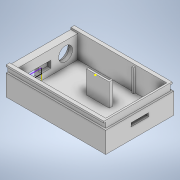
# Autodesk Inventor part: CajaArduinoNano
Saved by Autodesk Inventor 2021 (Build 250183000, 183)
## iProperties
Created: 2020-09-05
Part Number: CajaArduinoNano
Material: Genérico
Document SubType Name: Modeling
Designer: igtw1
Density: 1 g/cm^3
Appearance: Valor por defecto
Author: igtw1
Autodesk Inventor part; units mm, degrees
ref_plane "YZ Plane" through (0, 0, 0) normal (1, 0, 0) x (0, 1, 0)
ref_plane "XZ Plane" through (0, 0, 0) normal (0, 1, 0) x (-1, 0, 0)
ref_plane "XY Plane" through (0, 0, 0) normal (0, 0, 1) x (1, 0, 0)
sketch "Boceto1" plane through (0, 0, 0) normal (0, 1, 0) x (-1, 0, 0)
  line L0 (27.5, -17.5) -> (-27.5, -17.5)
  line L1 (-27.5, -17.5) -> (-27.5, 17.5)
  line L2 (-27.5, 17.5) -> (27.5, 17.5)
  line L3 (27.5, 17.5) -> (27.5, -17.5)
  line L4 (27.5, -17.5) -> (-27.5, 17.5) construction
  line L5 (-27.5, -17.5) -> (27.5, 17.5) construction
  point P0 (0, 0)
  dimension "d0" = 55
  dimension "d1" = 35
  constraints: 12 end point, 2 midpoint, 2 parallel, 1 horizontal, 1 perpendicular
  measures "d0" distance of L1.end L2.end
  measures "d1" distance of L0.end L1.end
extrude "Extrusión1" add sketch "Boceto1" along normal blind 15
sketch "Boceto2" plane through (0, 15, 0) normal (0, 1, 0) x (1, 0, 0)
  line L0 (25.5, -15.5) -> (-25.5, -15.5)
  line L1 (-25.5, -15.5) -> (-25.5, 15.5)
  line L2 (-25.5, 15.5) -> (25.5, 15.5)
  line L3 (25.5, 15.5) -> (25.5, -15.5)
  line L4 (25.5, -15.5) -> (-25.5, 15.5) construction
  line L5 (-25.5, -15.5) -> (25.5, 15.5) construction
  point P0 (0, 0)
  dimension "d4" = 51
  dimension "d5" = 31
  constraints: 12 end point, 2 midpoint, 2 parallel, 1 horizontal, 1 perpendicular
  measures "d4" distance of L1.end L2.end
  measures "d5" distance of L0.end L1.end
extrude "Extrusión2" cut sketch "Boceto2" against normal blind 13
sketch "Boceto3" plane through (-27.5, 0, -17.5) normal (-1, 0, 0) x (0, 0, 1)
  point P0 (17.5, 0)
sketch "Boceto4" plane through (0, 15, 0) normal (0, 1, 0) x (1, 0, 0)
  line L0 (-27.5, 17.5) -> (-27.5, -17.5) projected
  line L1 (-27.5, -17.5) -> (-29.5, -17.5)
  line L2 (-29.5, -17.5) -> (-29.5, 17.5)
  line L3 (-29.5, 17.5) -> (-27.5, 17.5)
  line L4 (-27.5, 17.5) -> (-27.5, -17.5)
  point P0 (0, 0)
  dimension "d8" = 2
  constraints: 8 end point, 2 parallel, 1 horizontal, 1 perpendicular
  measures "d8" distance of L2.end L3.end
extrude "Extrusión3" add sketch "Boceto4" against normal blind 15
sketch "Boceto5" plane through (-29.5, 15, -17.5) normal (-1, 0, 0) x (0, 0, 1)
  line L0 (35, 0) -> (0, 0) projected
  line L1 (0, 0) -> (9, 0)
  line L2 (9, 0) -> (9, -6.5)
  line L3 (2, -13) -> (33, -13) projected
  circle A0 centre (9, -6.5) radius 5.5
  point P0 (17.5, -15)
  dimension "d11" = 9
  dimension "d12" = 6.5
  dimension "d13" = 11
  constraints: 4 end point, 1 centre point, 1 coincident, 1 perpendicular, 1 point on line
  measures "d11" distance of L0.end L1.end
  measures "d12" distance of L1.end L2.end
  measures "d13" diameter of A0
extrude "Extrusión4" cut sketch "Boceto5" against normal blind 2
sketch "Boceto6" plane through (-27.5, 8.5, -8.5) normal (-1, 0, 0) x (0, 0, 1)
  circle A0 centre (0, 0) radius 4
  point P0 (8.5, -8.5)
  dimension "d16" = 8
  constraints: 1 centre point
  measures "d16" diameter of A0
extrude "Extrusión5" cut sketch "Boceto6" against normal blind 2
sketch "Boceto7" plane through (0, 2, 0) normal (0, 1, 0) x (1, 0, 0)
  line L0 (-27.5, 3) -> (-27.5, 14) projected
  line L1 (-27.5, 3) -> (-27.5, 8.5)
  line L2 (-25.5, -15.5) -> (-25.5, 15.5) projected
  line L3 (-25.5, 8.5) -> (-25.5, 1.5)
  line L4 (-25.5, 15.5) -> (25.5, 15.5) projected
  line L5 (7.5, 15.5) -> (7.5, 14.5)
  line L6 (7.5, 14.5) -> (6.5, 14.5)
  line L7 (6.5, 14.5) -> (6.5, 15.5)
  line L8 (6.5, 1.5) -> (6.5, 2.5547)
  line L9 (6.5, 2.5547) -> (7.5, 2.5547)
  line L10 (7.5, 2.5547) -> (7.5, 0.5)
  line L11 (7.5, 0.5) -> (-5.5, 0.5)
  line L12 (-5.5, 0.5) -> (-5.5, 1.5)
  line L13 (-5.5, 1.5) -> (6.5, 1.5)
  point P0 (0, 0)
  dimension "d19" = 7
  dimension "d27" = 32
  constraints: 22 end point, 4 point on line, 3 horizontal, 2 perpendicular, 1 midpoint
  measures "d19" distance of L3.start L3.end
  measures "d27" distance of L3.end L8.start
extrude "Extrusión6" add sketch "Boceto7" along normal blind 13 contours L8 L9 L10 L11 L12 L13
sketch "Boceto8" plane through (0, 2, 0) normal (0, 1, 0) x (1, 0, 0)
  line L0 (6.5, 1.5) -> (6.5, 2.5547) projected
  line L1 (-25.5, 15.5) -> (25.5, 15.5) projected
  line L2 (6.5, 15.5) -> (6.5, 14.5)
  line L3 (6.5, 14.5) -> (7.5, 14.5)
  line L4 (7.5, 14.5) -> (7.5, 15.5)
  point P0 (0, 0)
  constraints: 6 end point, 2 perpendicular, 1 point on line
extrude "Extrusión7" add sketch "Boceto8" along normal blind 13
sketch "Boceto9" plane through (0, 15, 0) normal (0, 1, 0) x (1, 0, 0)
  line L0 (-29.5, -17.5) -> (27.5, -17.5) projected
  line L1 (27.5, -17.5) -> (27.5, -21.5)
  line L2 (27.5, -21.5) -> (-29.5, -21.5)
  line L3 (-29.5, -21.5) -> (-29.5, -17.5)
  point P0 (0, 0)
  dimension "d34" = 4
  constraints: 6 end point, 2 perpendicular, 1 vertical
  measures "d34" distance of L0.end L1.end
extrude "Extrusión8" add sketch "Boceto9" against normal blind 15
sketch "Boceto10" plane through (0, 15, 0) normal (0, 1, 0) x (1, 0, 0)
  line L0 (25.5, -15.5) -> (-25.5, -15.5) projected
  line L1 (-25.5, -15.5) -> (25.5, -15.5)
  line L2 (25.5, -15.5) -> (25.5, -19.5)
  line L3 (25.5, -19.5) -> (-25.5, -19.5)
  line L4 (-25.5, -19.5) -> (-25.5, -15.5)
  point P0 (0, 0)
  dimension "d37" = 4
  constraints: 8 end point, 2 parallel, 1 horizontal, 1 perpendicular
  measures "d37" distance of L1.end L2.end
extrude "Extrusión9" cut sketch "Boceto10" against normal blind 13
sketch "Boceto11" plane through (-29.5, 0, -17.5) normal (-1, 0, 0) x (0, 0, 1)
  line L0 (39, 15) -> (37, 15)
  line L1 (39, 15) -> (0, 15) projected
  line L2 (37, 15) -> (27, 15)
  line L3 (0, 0) -> (39, 0) projected
  line L4 (2, 2) -> (37, 2) projected
  line L5 (27, 5.5) -> (27, 8.5)
  line L6 (27, 5.5) -> (31, 5.5)
  line L7 (31, 5.5) -> (31, 2.5)
  line L8 (31, 2.5) -> (23, 2.5)
  line L9 (23, 2.5) -> (23, 5.5)
  line L10 (23, 5.5) -> (27, 5.5)
  point P0 (17.5, 0)
  dimension "d41" = 10
  dimension "d45" = 3
  dimension "d46" = 4
  constraints: 16 end point, 4 perpendicular, 3 point on line, 1 horizontal
  measures "d41" distance of L0.end L2.end
  measures "d45" distance of L5.start L5.end
  measures "d46" distance of L5.start L6.end
extrude "Extrusión10" cut sketch "Boceto11" against normal blind 4
sketch "Boceto12" plane through (-25.5, 2, -15.5) normal (1, 0, 0) x (0, 0, -1)
  line L0 (-29, 3.5) -> (-29, 0.5) projected
  line L1 (-29, 3.5) -> (-25, 3.5)
  line L2 (-29, 3.5) -> (-21, 3.5) projected
  line L3 (-25, 6.5) -> (-21, 6.5)
  line L4 (-21, 0.5) -> (-21, 3.5) projected
  line L5 (-21, 6.5) -> (-21, 3.5)
  line L6 (-21, 3.5) -> (-29, 3.5)
  line L7 (-29, 6.5) -> (-29, 3.2703)
  line L8 (-29, 6.5) -> (-25, 6.5)
  point P0 (-15.5, -2)
  constraints: 12 end point, 3 collinear, 1 midpoint, 1 point on line, 1 vertical
sketch "Boceto13" plane through (-25.5, 2, -15.5) normal (1, 0, 0) x (0, 0, -1)
  line L0 (-25, 3.524) -> (-34.5, 3.524)
  line L1 (-35, 13) -> (-35, 0) projected
  line L2 (-34.5, 3.524) -> (-34.5, 6.524)
  line L3 (-35, 13) -> (0, 13) projected
  line L4 (-34.5, 6.524) -> (-15.5, 6.524)
  line L5 (-15.5, 6.524) -> (-15.5, 3.524)
  line L6 (-35, 0) -> (0, 0) projected
  line L7 (-15.5, 3.524) -> (-25, 3.524)
  point P0 (-15.5, -2)
  dimension "d52" = 9.5
  dimension "d54" = 3
  dimension "d55" = 19
  dimension "d56" = 3
  constraints: 10 end point, 3 perpendicular, 1 horizontal
  measures "d52" distance of L0.start L0.end
  measures "d54" distance of L0.end L2.end
  measures "d55" distance of L2.end L4.end
  measures "d56" distance of L4.end L5.end
extrude "Extrusión11" cut sketch "Boceto13" against normal blind 2
sketch "Boceto14" plane through (27.5, 0, -17.5) normal (1, 0, 0) x (0, 0, -1)
  line L0 (0, 15) -> (0, 0) projected
  line L1 (0, 0) -> (-19.5, 0)
  line L2 (-39, 0) -> (0, 0) projected
  line L3 (-19.5, 0) -> (-19.5, 7.5)
  line L4 (-36.5, 8.524) -> (-17.5, 8.524) projected
  line L5 (-19.5, 7.5) -> (-24.5, 7.5)
  line L6 (-39, 15) -> (-39, 0) projected
  line L7 (-24.5, 7.5) -> (-24.5, 6.5)
  line L8 (-24.5, 6.5) -> (-14.5, 6.5)
  line L9 (-14.5, 6.5) -> (-14.5, 8.5)
  line L10 (-37, 15) -> (-2, 15) projected
  line L11 (-24.5, 6.5) -> (-24.5, 8.5)
  line L12 (-24.5, 8.5) -> (-14.5, 8.5)
  point P0 (-17.5, 0)
  dimension "d59" = 19.5
  dimension "d60" = 7.5
  dimension "d61" = 5
  dimension "d62" = 1
  dimension "d63" = 10
  dimension "d64" = 2
  dimension "d65" = 2
  constraints: 16 end point, 4 perpendicular, 1 horizontal, 1 midpoint, 1 vertical
  measures "d59" distance of L0.end L1.end
  measures "d60" distance of L1.end L3.end
  measures "d61" distance of L3.end L5.end
  measures "d62" distance of L5.end L7.end
  measures "d63" distance of L7.end L8.end
  measures "d64" distance of L8.end L9.end
  measures "d65" distance of L7.end L11.end
extrude "Extrusión12" cut sketch "Boceto14" against normal blind 3
sketch "Boceto15" plane through (0, 15, 0) normal (0, 1, 0) x (1, 0, 0)
  line L0 (27.5, -21.5) -> (-29.5, -21.5) projected
  line L1 (27.5, 17.5) -> (-29.5, 17.5) projected
  line L2 (-29.5, -21.5) -> (27.5, -21.5)
  line L3 (27.5, -21.5) -> (27.5, 17.5)
  line L4 (27.5, 17.5) -> (-29.5, 17.5)
  line L5 (27.5, -21.5) -> (27.5, 17.5) projected
  line L6 (27.5, 17.5) -> (27.5, 16.5)
  line L7 (26.5, 16.5) -> (-28.5, 16.5)
  line L8 (-28.5, -20.5) -> (26.5, -20.5)
  line L9 (26.5, -20.5) -> (26.5, 16.5)
  line L10 (-28.5, 16.5) -> (-29.5, 16.5)
  line L11 (-29.5, 17.5) -> (-29.5, -21.5) projected
  line L12 (27.5, 17.5) -> (-29.5, 17.5) projected
  line L13 (-29.5, 16.5) -> (-29.5, 17.5)
  line L14 (-28.5, -20.5) -> (-29.5, -20.5)
  line L15 (-29.5, -21.5) -> (-29.5, -20.5)
  point P0 (0, 0)
  dimension "d69" = 1
  dimension "d70" = 55
  dimension "d71" = 37
  constraints: 22 end point, 3 horizontal, 3 point on line, 2 parallel, 2 perpendicular, 1 collinear, 1 vertical
  measures "d69" distance of L6.end L7.start
  measures "d70" distance of L8.end L8.start
  measures "d71" distance of L8.start L7.end
sketch "Boceto16" plane through (0, 15, 0) normal (0, 1, 0) x (1, 0, 0)
  point P0 (0, 0)
extrude "Extrusión13" cut sketch "Boceto15" against normal blind 3 contours L0 L11 L14 L8 L9 L7 L10 L1 L3
sketch "Boceto17" plane through (-29.5, 15, 20.5) normal (0, 0, 1) x (1, 0, 0)
  line L0 (0, 0) -> (56, 0) projected
  line L1 (56, 0) -> (56, -3) projected
  line L2 (0, 0) -> (56, 0)
  line L3 (56, 0) -> (56, -1.5)
  line L4 (56, -1.5) -> (0, -1.5)
  line L5 (0, -1.5) -> (0, 0)
  point P0 (29.5, -15)
  constraints: 8 end point, 2 parallel, 1 horizontal, 1 midpoint, 1 perpendicular
extrude "Extrusión14" add sketch "Boceto17" along normal blind 1
sketch "Boceto18" plane through (26.5, 15, -16.5) normal (0, 0, -1) x (-1, 0, 0)
  line L0 (0, 0) -> (56, 0) projected
  line L1 (0, -1.5) -> (56, -1.5) projected
  line L2 (0, 0) -> (56, 0)
  line L3 (56, 0) -> (56, -1.5)
  line L4 (56, -1.5) -> (0, -1.5)
  line L5 (0, -1.5) -> (0, 0)
  point P0 (26.5, -15)
  constraints: 8 end point, 2 parallel, 1 horizontal, 1 perpendicular
extrude "Extrusión15" add sketch "Boceto18" along normal blind 1
sketch "Boceto19" plane through (-29.5, 0, -17.5) normal (-1, 0, 0) x (0, 0, 1)
  line L0 (23, 2.5) -> (23, 5.5) projected
  line L1 (23, 5.5) -> (31, 5.5)
  line L2 (31, 5.5) -> (31, 8.5)
  line L3 (31, 8.5) -> (23, 8.5)
  line L4 (23, 8.5) -> (23, 5.5)
  point P0 (17.5, 0)
  dimension "d78" = 8
  dimension "d79" = 3
  constraints: 8 end point, 2 parallel, 1 horizontal, 1 perpendicular
  measures "d78" distance of L3.end L2.end
  measures "d79" distance of L2.end L1.end
extrude "Extrusión16" cut sketch "Boceto19" against normal blind 6
sketch "Boceto20" plane through (-29.5, 0, -17.5) normal (-1, 0, 0) x (0, 0, 1)
  line L0 (23, 8.5) -> (23, 5.524) projected
  line L1 (23, 8.5) -> (22.5, 8.5)
  line L2 (24.5, 8.5) -> (14.5, 8.5) projected
  line L3 (22.5, 8.5) -> (22.5, 2.5)
  line L4 (22.5, 2.5) -> (31.5, 2.5)
  line L5 (23, 2.5) -> (31, 2.5) projected
  line L6 (31.5, 2.5) -> (31.5, 8.5)
  line L7 (31.5, 8.5) -> (22.5, 8.5)
  point P0 (17.5, 0)
  dimension "d82" = 0.5
  dimension "d83" = 6
  dimension "d84" = 9
  dimension "d85" = 6
  constraints: 10 end point, 2 point on line, 1 collinear, 1 perpendicular
  measures "d82" distance of L0.start L1.end
  measures "d83" distance of L1.end L3.end
  measures "d84" distance of L3.end L4.end
  measures "d85" distance of L4.end L6.end
extrude "Extrusión17" cut sketch "Boceto20" against normal blind 6
sketch "Boceto21" plane through (-25.5, 2, -15.5) normal (1, 0, 0) x (0, 0, -1)
  line L0 (-34.5, 6.524) -> (-15.5, 6.524) projected
  line L1 (-34.5, 6.524) -> (-34.5, 7.524)
  line L2 (-34.5, 7.524) -> (-15.5, 7.524)
  line L3 (-15.5, 7.524) -> (-15.5, 6.524)
  line L4 (-15.5, 6.524) -> (-34.5, 6.524)
  point P0 (-15.5, -2)
  dimension "d88" = 1
  constraints: 8 end point, 3 perpendicular, 1 vertical
  measures "d88" distance of L0.start L1.end
extrude "Extrusión18" cut sketch "Boceto21" against normal blind 2
sketch "Boceto22" plane through (26.5, 12, 20.5) normal (1, 0, 0) x (0, 0, -1)
  line L0 (0, 0) -> (37, 0) projected
  line L1 (37, 0) -> (37, 3)
  line L2 (-1, 3) -> (38, 3) projected
  line L3 (37, 3) -> (38, 3)
  line L4 (37, 0) -> (38, 0) projected
  line L5 (38, 3) -> (38, 0)
  line L6 (38, 0) -> (37, 0)
  line L7 (0, 1.5) -> (0, 0) projected
  line L8 (-1, 0) -> (-1, -12) projected
  line L9 (0, 0) -> (-1, 0)
  line L10 (-1, 0) -> (-1, 3)
  line L11 (0, 3) -> (0, 0)
  point P0 (20.5, -12)
  constraints: 14 end point, 3 perpendicular, 2 horizontal, 2 point on line, 1 collinear, 1 vertical
extrude "Extrusión19" cut sketch "Boceto22" against normal blind 100 contours L9 L10 L2 L11 L7 | L1 L2 L5 L4
sketch "Boceto23" plane through (26.5, 15, 20.5) normal (1, 0, 0) x (0, 0, -1)
  line L0 (37, 0) -> (37, -3) projected
  line L1 (37, 0) -> (38, 0)
  line L2 (38, 0) -> (38.5, 0)
  line L3 (38.5, 0) -> (38.5, 1)
  line L4 (38.5, 1) -> (37, 1)
  line L5 (37, 1) -> (36, 1)
  line L6 (36, 1) -> (36, 0)
  line L7 (37, 0) -> (36, 0)
  line L8 (0, 0) -> (37, 0) projected
  point P0 (20.5, -15)
  dimension "d93" = 1
  dimension "d94" = 0.5
  dimension "d95" = 1
  constraints: 14 end point, 3 perpendicular, 2 horizontal, 1 collinear, 1 point on line
  measures "d93" distance of L0.start L1.end
  measures "d94" distance of L1.end L2.end
  measures "d95" distance of L2.end L3.end
extrude "Extrusión20" add sketch "Boceto23" against normal blind 56
sketch "Boceto24" plane through (26.5, 15, 20.5) normal (1, 0, 0) x (0, 0, -1)
  line L0 (36, 0) -> (0, 0) projected
  line L1 (0, 0) -> (-1.5, 0)
  line L2 (-1.5, 0) -> (-1.5, 1)
  line L3 (-1.5, 1) -> (0.5, 1)
  line L4 (0.5, 1) -> (1, 1)
  line L5 (1, 0) -> (36, 0) projected
  line L6 (1, 1) -> (1, 0)
  line L7 (1, 0) -> (0, 0)
  point P0 (20.5, -15)
  dimension "d98" = 1.5
  dimension "d99" = 1
  dimension "d100" = 2
  dimension "d101" = 0.5
  constraints: 12 end point, 2 perpendicular, 1 horizontal, 1 point on line
  measures "d98" distance of L0.end L1.end
  measures "d99" distance of L1.end L2.end
  measures "d100" distance of L2.end L3.end
  measures "d101" distance of L3.end L4.end
extrude "Extrusión21" add sketch "Boceto24" against normal blind 56
sketch "Boceto25" plane through (26.5, 15, 19.5) normal (1, 0, 0) x (0, 0, -1)
  line L0 (-2.5, 1) -> (0, 1) projected
  line L1 (-1, 0) -> (-2.5, 0) projected
  line L2 (-2.5, 1) -> (-2, 1)
  line L3 (-2, 1) -> (-2, 0)
  line L4 (-2, 0) -> (-2.5, 0)
  line L5 (-2.5, 0) -> (-2.5, 1)
  line L6 (37.5, 1) -> (35, 1) projected
  line L7 (36, 0) -> (37.5, 0) projected
  line L8 (37.5, 1) -> (37, 1)
  line L9 (37, 1) -> (37, 0)
  line L10 (37, 0) -> (37.5, 0)
  line L11 (37.5, 0) -> (37.5, 1)
  point P0 (19.5, -15)
  point P1 (-2, 1)
  dimension "d104" = 0.5
  dimension "d105" = 0.5
  constraints: 16 end point, 4 parallel, 2 horizontal, 2 perpendicular, 2 point on line
  measures "d104" distance of L3.end L4.end
  measures "d105" distance of L10.end L9.end
extrude "Extrusión22" cut sketch "Boceto25" against normal blind 56
sketch "Boceto26" plane through (26.5, 15, 19.5) normal (1, 0, 0) x (0, 0, -1)
  point P0 (19.5, -15)
sketch "Boceto27" plane through (26.5, 15, 19.5) normal (1, 0, 0) x (0, 0, -1)
  line L0 (35, 0) -> (0, 0) projected
  line L1 (0, 1) -> (0, 0) projected
  line L2 (35, 0) -> (0, 0)
  line L3 (0, 0) -> (0, 1)
  line L4 (0, 1) -> (35, 1)
  line L5 (35, 1) -> (35, 0)
  point P0 (19.5, -15)
  constraints: 8 end point, 2 parallel, 1 horizontal, 1 perpendicular
extrude "Extrusión23" add sketch "Boceto27" against normal blind 1
